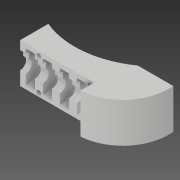
# Autodesk Inventor part: final lock housing back
Saved by Autodesk Inventor 2017 (Build 210142000, 142)
## iProperties
Created: 2018-04-20
Part Number: final lock housing back
Material: Generic
Document SubType Name: Modeling
Designer: natha
Density: 1 g/cm^3
Appearance: Default
Author: natha
Autodesk Inventor part; units mm, degrees
ref_plane "YZ Plane" through (0, 0, 0) normal (1, 0, 0) x (0, 1, 0)
ref_plane "XZ Plane" through (0, 0, 0) normal (0, 1, 0) x (-1, 0, 0)
sketch "Sketch1" plane through (0, 0, 0) normal (0, 0, 1) x (1, 0, 0)
  circle A0 centre (12.2387, 16.51) radius 2.54 projected
  line L0 (19.8587, 0) -> (0, 0) projected
  line L1 (19.8587, 0) -> (19.8587, 22.225) projected
  line L2 (0, 22.225) -> (19.8587, 22.225) projected
  line L3 (0, 0) -> (0, 22.225) projected
  line L4 (-42.016, 22.225) -> (-42.016, 0) projected
  line L5 (-42.016, 22.225) -> (19.8587, 22.225)
  line L6 (19.8587, 22.225) -> (19.8587, 0)
  line L7 (19.8587, 0) -> (-42.016, 0)
  line L8 (-42.016, 0) -> (-42.016, 22.225)
  constraints: 8 end point, 2 parallel, 1 horizontal, 1 perpendicular
ref_plane "Work Plane1" through (-48.366, 22.225, 28.1991) normal (0, 0, 1) x (1, 0, 0)
extrude "Extrusion1" add sketch "Sketch1" along normal up to surface (28.1991 mm away) contours A0 | L0 L3 L2 L1 | L7 L4 L5 L3
sketch "Sketch6" plane through (-42.016, 22.225, 0) normal (0, 1, 0) x (1, 0, 0)
  arc A0 (36.4747, -28.1991) -> (61.8747, -2.7991) centre (36.4747, -2.7991) ccw projected
  arc A1 (-11.8913, 0) -> (42.016, 0) centre (15.0623, 38.2739) ccw projected
  line L0 (0, -17.4041) -> (38.1, -17.4041)
  line L1 (0, 0) -> (0, -28.1991) projected
  line L2 (0, -6.049) -> (0, 0)
  line L3 (0, 0) -> (42.016, 0)
  line L4 (61.8747, 0) -> (61.8747, -28.1991) projected
  line L5 (61.8747, -2.7991) -> (61.8747, -28.1991)
  line L6 (61.8747, -28.1991) -> (36.4747, -28.1991)
  line L7 (38.1, -17.4041) -> (38.1, -28.147)
  line L8 (0, -17.4041) -> (0, -6.049)
  line L9 (61.8747, -28.1991) -> (0, -28.1991) projected
  line L10 (38.1, -28.1991) -> (36.4747, -28.1991)
  line L11 (38.1, -17.4041) -> (0, -17.4041)
  line L12 (0, -17.4041) -> (0, -28.1991)
  line L13 (0, -28.1991) -> (38.1, -28.1991)
  line L14 (38.1, -28.1991) -> (38.1, -17.4041)
  line L15 (0, -23.7541) -> (38.1, -23.7541)
  line L16 (0, -28.1991) -> (38.9215, -28.2018)
  line L17 (38.9215, -28.2018) -> (38.9212, -28.1991)
  line L18 (36.4747, -20.5791) -> (38.1, -20.5791)
  line L19 (36.4747, -20.5791) -> (0, -20.5791)
  constraints: 34 end point, 6 point on line, 5 perpendicular, 4 horizontal, 3 collinear, 3 point on circle, 2 parallel, 4 other
extrude "Extrusion6" cut sketch "Sketch6" against normal through all contours L9 L1 L15 L7 A0 | A0 L14 L6 | L6 L17 L16 L9 | L1 L3 A1 | A0 L4 L6 L14 | L15 L1 L19 L18 L7
sketch "Sketch7" plane through (-42.016, 0, 6.049) normal (-1, 0, 0) x (0, 0, 1)
  line L0 (16.1176, 18.669) -> (12.9426, 18.669) projected
  circle A0 centre (14.5301, 10.922) radius 3.175 projected
  arc A1 (12.8156, 13.744) -> (16.2446, 13.744) centre (14.5301, 10.922) ccw
  line L1 (16.2446, 18.796) -> (16.2446, 10.795)
  line L2 (16.2446, 10.795) -> (12.8156, 10.795)
  line L3 (12.8156, 10.795) -> (12.8156, 18.796)
  line L4 (12.8156, 17.399) -> (16.2446, 17.399)
  point P0 (-6.049, 0)
  dimension "d31" = 6.604
  dimension "d35" = 6.477
  constraints: 8 end point, 4 point on line, 2 point on circle, 1 centre point, 1 coincident, 1 horizontal, 1 parallel, 1 perpendicular
  measures "d31" diameter of A1
  measures "d35" distance from line of L4 A0.centre
extrude "Extrusion7" cut sketch "Sketch7" against normal blind 38.1
sketch "Sketch8" plane through (-42.016, 0, 20.5791) normal (0, 0, 1) x (1, 0, 0)
  line L0 (0, 14.097) -> (33.655, 14.097)
  line L1 (38.1, 7.62) -> (0, 7.62) projected
  line L2 (0, 14.097) -> (0, 7.62)
  line L3 (0, 13.744) -> (38.1, 13.744) projected
  line L4 (0, 22.225) -> (0, 0) projected
  line L5 (38.1, 10.8585) -> (0, 10.8585)
  line L6 (9.525, 13.6716) -> (5.08, 13.6716) projected
  line L7 (9.525, 13.6716) -> (9.525, 17.272) projected
  line L8 (9.525, 17.272) -> (5.08, 17.272) projected
  line L9 (5.08, 17.272) -> (5.08, 13.6716) projected
  line L10 (19.05, 13.6716) -> (14.605, 13.6716) projected
  line L11 (19.05, 13.6716) -> (19.05, 17.272) projected
  line L12 (19.05, 17.272) -> (14.605, 17.272) projected
  line L13 (14.605, 17.272) -> (14.605, 13.6716) projected
  line L14 (28.575, 13.6716) -> (24.13, 13.6716) projected
  line L15 (28.575, 13.6716) -> (28.575, 17.272) projected
  line L16 (28.575, 17.272) -> (24.13, 17.272) projected
  line L17 (24.13, 17.272) -> (24.13, 13.6716) projected
  line L18 (38.1, 13.6716) -> (33.655, 13.6716) projected
  line L19 (38.1, 13.6716) -> (38.1, 17.272) projected
  line L20 (38.1, 17.272) -> (33.655, 17.272) projected
  line L21 (33.655, 17.272) -> (33.655, 13.6716) projected
  line L22 (0, 10.8585) -> (5.08, 10.8585)
  line L23 (5.08, 10.8585) -> (5.08, 19.7485)
  line L24 (5.08, 19.7485) -> (0, 19.7485)
  line L25 (0, 19.7485) -> (0, 10.8585)
  line L26 (9.525, 10.8585) -> (14.605, 10.8585)
  line L27 (14.605, 10.8585) -> (14.605, 19.7485)
  line L28 (14.605, 19.7485) -> (9.525, 19.7485)
  line L29 (9.525, 19.7485) -> (9.525, 10.8585)
  line L30 (19.05, 19.7485) -> (24.13, 19.7485)
  line L31 (24.13, 19.7485) -> (24.13, 10.8585)
  line L32 (24.13, 10.8585) -> (19.05, 10.8585)
  line L33 (19.05, 10.8585) -> (19.05, 19.7485)
  line L34 (28.575, 10.8585) -> (33.655, 10.8585)
  line L35 (33.655, 10.8585) -> (33.655, 19.7485)
  line L36 (33.655, 19.7485) -> (28.575, 19.7485)
  line L37 (28.575, 19.7485) -> (28.575, 10.8585)
  point P0 (42.016, 0)
  dimension "d36" = 8.89
  constraints: 38 end point, 8 parallel, 7 point on line, 5 horizontal, 5 perpendicular, 2 other
  measures "d36" distance of L23.end L22.end
revolve "Revolution2" cut sketch "Sketch8" angle 360 about axis through (-3.916, 10.8585, 20.5791) along (-1, 0, 0) contours L4 L24 L23 L9 L0 | L0 L9 L3 L2 | L3 L9 L23 L5 L2 | L7 L29 L28 L27 L13 L0 | L0 L13 L3 L7 | L3 L13 L27 L5 L29 L7 | L11 L33 L30 L31 L17 L0 | L0 L17 L3 L11 | L3 L17 L31 L5 L33 L11 | L15 L37 L36 L35 L21 L0 | L0 L21 L3 L15 | L3 L21 L35 L5 L37 L15
sketch "Sketch9" plane through (-42.016, 22.225, 20.5791) normal (0, 0, 1) x (1, 0, 0)
  line L0 (19.05, -4.826) -> (19.05, -2.4765) projected
  line L1 (19.05, -2.4765) -> (24.13, -2.4765) projected
  line L2 (24.13, -2.4765) -> (24.13, -4.826) projected
  line L3 (24.13, -4.826) -> (28.575, -4.826) projected
  line L4 (28.575, -4.826) -> (28.575, -2.4765) projected
  line L5 (28.575, -2.4765) -> (33.655, -2.4765) projected
  line L6 (33.655, -2.4765) -> (33.655, -4.826) projected
  line L7 (33.655, -4.826) -> (38.1, -4.826) projected
  line L8 (38.1, 0) -> (38.1, -4.826) projected
  line L9 (0, 0) -> (38.1, 0) projected
  line L10 (0, -2.4765) -> (0, 0) projected
  line L11 (0, -2.4765) -> (5.08, -2.4765) projected
  line L12 (5.08, -2.4765) -> (5.08, -4.826) projected
  line L13 (5.08, -4.826) -> (9.525, -4.826) projected
  line L14 (9.525, -4.826) -> (9.525, -2.4765) projected
  line L15 (9.525, -2.4765) -> (14.605, -2.4765) projected
  line L16 (14.605, -2.4765) -> (14.605, -4.826) projected
  line L17 (14.605, -4.826) -> (19.05, -4.826) projected
  circle A0 centre (7.3025, -2.4765) radius 1.27
  line L18 (19.05, -20.2565) -> (19.05, -14.605) projected
  line L19 (19.05, -14.605) -> (14.605, -14.605) projected
  line L20 (14.605, -14.605) -> (14.605, -20.2565) projected
  line L21 (14.605, -20.2565) -> (9.525, -20.2565) projected
  line L22 (9.525, -20.2565) -> (9.525, -14.605) projected
  line L23 (9.525, -14.605) -> (5.08, -14.605) projected
  line L24 (5.08, -14.605) -> (5.08, -20.2565) projected
  line L25 (5.08, -20.2565) -> (0, -20.2565) projected
  line L26 (0, -22.225) -> (0, -20.2565) projected
  line L27 (38.1, -22.225) -> (0, -22.225) projected
  line L28 (38.1, -14.605) -> (38.1, -22.225) projected
  line L29 (38.1, -14.605) -> (33.655, -14.605) projected
  line L30 (33.655, -14.605) -> (33.655, -20.2565) projected
  line L31 (33.655, -20.2565) -> (28.575, -20.2565) projected
  line L32 (28.575, -20.2565) -> (28.575, -14.605) projected
  line L33 (28.575, -14.605) -> (24.13, -14.605) projected
  line L34 (24.13, -14.605) -> (24.13, -20.2565) projected
  line L35 (24.13, -20.2565) -> (19.05, -20.2565) projected
  circle A1 centre (35.8775, -20.2565) radius 1.27
  circle A2 centre (35.8775, -2.4765) radius 1.27
  circle A3 centre (7.3025, -20.2565) radius 1.27
  point P0 (42.016, -22.225)
  dimension "d38" = 2.54
  dimension "d39" = 2.54
  dimension "d40" = 2.54
  dimension "d41" = 2.54
  constraints: 4 centre point
  measures "d38" diameter of A0
  measures "d39" diameter of A1
  measures "d40" diameter of A2
  measures "d41" diameter of A3
extrude "Extrusion8" cut sketch "Sketch9" against normal blind 6.35 contours A0 | A1 | A2 | A3
sketch "Sketch10" plane through (0, 22.225, 0) normal (0, 1, 0) x (1, 0, 0)
  arc A0 (-42.016, -6.049) -> (0, 0) centre (-26.9537, 38.2739) ccw projected
  line L0 (-42.016, -6.049) -> (-42.016, -20.5791) projected
  line L1 (-42.016, -20.5791) -> (-3.916, -20.5791) projected
  line L2 (-3.916, -20.5791) -> (-3.916, -28.147) projected
  arc A1 (-3.916, -28.147) -> (19.8587, -2.7991) centre (-5.5413, -2.7991) ccw projected
  line L3 (19.8587, 0) -> (19.8587, -2.7991) projected
  line L4 (19.8587, 0) -> (0, 0) projected
  line L5 (0, 0) -> (19.8587, 0) projected
  arc A2 (-45.191, -4.8398) -> (0, 0) centre (-26.9537, 38.2739) ccw
  line L6 (-42.016, -20.5791) -> (-45.191, -20.5791)
  line L7 (-45.191, -20.5791) -> (-45.191, -4.8398)
  line L8 (-42.016, -6.049) -> (-42.016, -20.5791)
  constraints: 6 end point, 3 point on circle, 1 centre point, 1 coincident, 1 horizontal, 1 parallel, 1 perpendicular
extrude "Extrusion9" add sketch "Sketch10" against normal up to surface (22.225 mm away) contours L0 L6 L7 A2
sketch "Sketch11" plane through (-36.936, 1.9685, 20.5791) normal (-1, 0, 0) x (0, 0, 1)
  line L0 (-1.7145, 15.4305) -> (0, 15.4305) projected
  line L1 (0, 19.05) -> (0, 16.51) projected
  line L2 (0, 20.2565) -> (0, 15.4305) projected
  line L3 (7.5679, 20.2565) -> (-17.78, 20.2565) projected
  line L4 (-1.7145, 11.7755) -> (-1.7145, 15.4305) projected
  arc A0 (-1.7145, 11.7755) -> (0, 5.6515) centre (0, 8.9535) ccw projected
  line L5 (0, 0) -> (0, 5.6515) projected
  line L6 (0, 1.27) -> (0, -1.27) projected
  line L7 (0, 5.6515) -> (0, -1.9685) projected
  arc A1 (0, 17.78) -> (0, 0) centre (0, 8.89) ccw projected
  line L8 (-1.7145, 15.4305) -> (0, 15.4305) projected
  line L9 (0, 15.4305) -> (0, 5.6515)
  point P0 (-20.5791, -1.9685)
  constraints: 2 end point, 1 collinear
extrude "Extrusion10" cut sketch "Sketch11" along normal through all contours L0 L9 A0 L4
sketch "Sketch12" plane through (0, 0, 0) normal (0, 0, -1) x (-1, 0, 0)
  circle A0 centre (-12.2387, 16.51) radius 2.54
  circle A1 centre (-12.2387, 16.51) radius 2.54
  line L0 (0.9001, 2.794) -> (-17.0647, 2.794)
  line L1 (0.9001, 2.794) -> (0.9001, 22.225)
  line L2 (-17.0647, 22.225) -> (0.9001, 22.225)
  line L3 (-17.0647, 2.794) -> (-17.0647, 22.225)
  line L4 (60.812, 2.794) -> (60.812, 18.669)
  line L5 (60.812, 18.669) -> (51.9355, 18.669)
  line L6 (51.9355, 18.669) -> (51.9355, 2.794)
  line L7 (70.972, 2.794) -> (60.812, 2.794)
  line L8 (-17.0647, 2.794) -> (-6.9047, 2.794)
  line L9 (-6.9047, 2.794) -> (-6.9047, 19.939)
  line L10 (-6.9047, 19.939) -> (-17.0647, 19.939)
  line L11 (-17.0647, 19.939) -> (-17.0647, 2.794)
  line L12 (3.916, 0) -> (3.916, 22.225)
  point P0 (0, 0)
revolve "Revolution3" cut sketch "Sketch12" angle 80 about axis through (-3.916, 0, 0) along (0, -1, 0) contours A0 | L0 L3 L10 L9
sketch "Sketch13" plane through (6.9047, 19.939, 0) normal (0, -1, 0) x (1, 0, 0)
  arc A0 (10.16, 0) -> (-7.1774, 20.6619) centre (-10.8207, 0) ccw projected
  line L0 (-8.9417, 10.6563) -> (-7.1774, 20.6619) projected
  arc A1 (0, 0) -> (-8.9417, 10.6563) centre (-10.8207, 0) ccw projected
  arc A2 (-2.5072, 15.3858) -> (-4.0166, 12.5925) centre (-3.2619, 13.9892) ccw
  arc A3 (-5.6768, 9.5199) -> (-8.9417, 10.6563) centre (-10.8207, 0) ccw
  arc A4 (-0.847, 18.4585) -> (-7.1774, 20.6619) centre (-10.8207, 0) ccw
  line L1 (-7.1774, 20.6619) -> (-8.9417, 10.6563)
  arc A5 (-0.847, 18.4585) -> (-8.0596, 15.6591) centre (-3.2619, 13.9892) ccw
  arc A6 (-8.3414, 14.0608) -> (-5.6768, 9.5199) centre (-3.2619, 13.9892) ccw
  arc A7 (-0.847, 18.4585) -> (-8.0596, 15.6591) centre (-3.2619, 13.9892) ccw
  arc A8 (-8.3414, 14.0608) -> (-5.6768, 9.5199) centre (-3.2619, 13.9892) ccw
  arc A9 (6.6675, 0) -> (-2.5072, 15.3858) centre (-10.8207, 0) ccw
  arc A10 (3.4925, 0) -> (-4.0166, 12.5925) centre (-10.8207, 0) ccw
  line L2 (6.6675, 0) -> (3.4925, 0)
  line L3 (-6.9047, 0) -> (12.954, 0) projected
  dimension "d52" = 3.175
  constraints: 20 point on circle, 9 centre point, 5 coincident, 4 end point, 2 collinear, 1 midpoint, 1 point on line
  measures "d52" diameter of A2
extrude "Extrusion11" add sketch "Sketch13" along normal up to next contours A5 L0 A0 | L2 A10 A2 A9 | A6 A1 L0
chamfer "Chamfer1" [suppressed]
fillet "Fillet1" [suppressed]
fillet "Fillet2" [suppressed]
body "Solid1"
